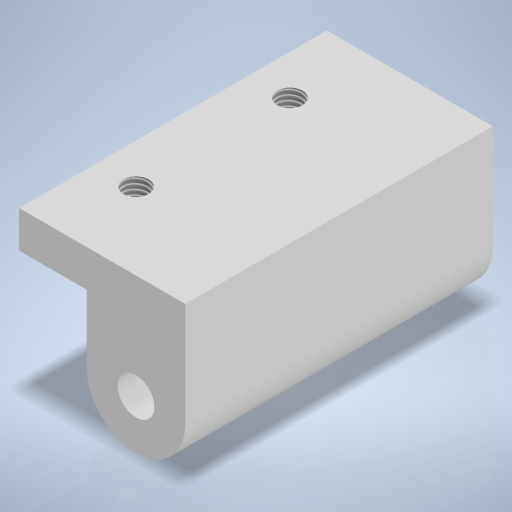
# Autodesk Inventor part: 103
Saved by Autodesk Inventor 2024 (Build 280153000, 153)
## iProperties
Created: 2024-06-11
Part Number: 103
Material: Generisch
Document SubType Name: Modeling
Designer: ffogue
Density: 1 g/cm^3
Appearance: Vorgabe
Author: ffogue
Autodesk Inventor part; units mm, degrees
ref_plane "YZ Plane" through (0, 0, 0) normal (1, 0, 0) x (0, 1, 0)
ref_plane "XZ Plane" through (0, 0, 0) normal (0, 1, 0) x (-1, 0, 0)
ref_plane "XY Plane" through (0, 0, 0) normal (0, 0, 1) x (1, 0, 0)
sketch "Skizze1" plane through (0, 0, 0) normal (0, 1, 0) x (-1, 0, 0)
  arc A0 (-8, 0) -> (8, 0) centre (0, 0) ccw
  line L0 (8, 0) -> (8, 11)
  line L1 (8, 17) -> (-8, 17)
  line L2 (-8, 17) -> (-8, 0)
  line L3 (8, 17) -> (19, 17)
  line L4 (19, 17) -> (19, 11)
  line L5 (19, 11) -> (8, 11)
  dimension "d0" = 16
  dimension "d1" = 16
  dimension "d2" = 6
  dimension "d3" = 19
  dimension "d4" = 11
  dimension "d5" = 17
  constraints: 12 end point, 4 perpendicular, 2 point on circle, 1 centre point, 1 coincident, 1 horizontal, 1 vertical
  measures "d0" diameter of A0
  measures "d1" distance between parallel lines of L2 L0
  measures "d2" distance between parallel lines of L5 L3
  measures "d3" distance from line of L4 point (0, 0)
  measures "d4" distance of L4.end L0.end
  measures "d5" distance from line of point (0, 0) L1
extrude "Extrusion1" add sketch "Skizze1" along normal blind 50
sketch "Skizze2" plane through (0, 50, 0) normal (0, 1, 0) x (1, 0, 0)
  arc A0 (8, 0) -> (-8, 0) centre (0, 0) ccw projected
  constraints: 1 coincident
hole "Bohrung1" at (0, 50, 0) direction (0, -1, 0) diameter 6 end through all
sketch "Skizze3" plane through (-19, 0, 11) normal (-1, 0, 0) x (0, 0, 1)
  line L0 (0, 0) -> (0, 50) projected
  line L1 (0, 31) -> (-11, 31)
  arc A0 (-11, 31) -> (-11, 19) centre (-11, 25) ccw
  line L2 (-11, 19) -> (0, 19)
  line L3 (0, 31) -> (0, 19)
  point P0 (-11, 0)
  point P1 (0, 25)
  dimension "d15" = 6
  constraints: 6 end point, 2 point on circle, 2 point on line, 2 tangent, 1 centre point, 1 horizontal, 1 horizontal alignment, 1 midpoint, 1 parallel, 1 perpendicular, 1 vertical alignment
  measures "d15" radius of A0
extrude "Extrusion2" add sketch "Skizze3" against normal up to surface (11 mm away)
sketch "Skizze4" plane through (-19, 0, 11) normal (-1, 0, 0) x (0, 0, 1)
  arc A0 (-11, 31) -> (-11, 19) centre (-11, 25) ccw projected
  point P0 (-11, 0)
  constraints: 1 coincident
hole "Bohrung2" at (-19, 25, 0) direction (1, 0, 0) diameter 9 depth 11
sketch "Skizze5" plane through (-8, 50, 11) normal (0, 0, -1) x (-1, 0, 0)
  line L0 (11, -19) -> (11, 0) projected
  line L1 (11, -31) -> (11, -19) projected
  point P0 (-8, -50)
  point P1 (4.5, -12.5)
  point P2 (4.5, -37.5)
  point P3 (11, -25)
  dimension "d32" = 6.5
  dimension "d33" = 12.5
  dimension "d34" = 25
  constraints: 1 midpoint, 1 vertical alignment
  measures "d32" distance from line of point (4.5, -12.5) L0
  measures "d33" vertical distance of point (11, -25) point (4.5, -12.5)
  measures "d34" distance of point (4.5, -37.5) point (4.5, -12.5)
hole "Bohrung3" at (-12.5, 37.5, 11) at (-12.5, 12.5, 11) direction (0, 0, 1) diameter 4.134 end through all thread size "M5x0.8" class "6H" standard "ISO Metric profile"
